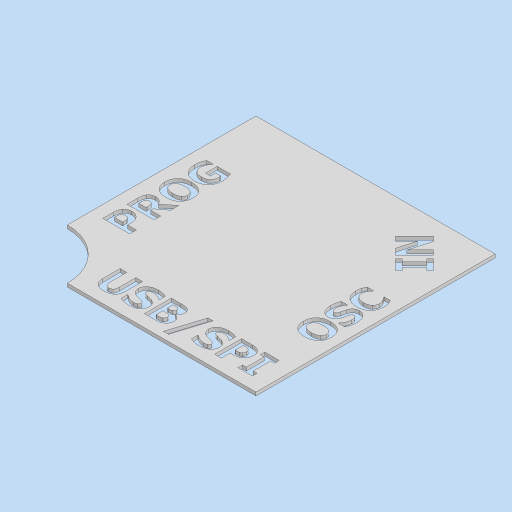
# Autodesk Inventor part: mcu_label
Saved by Autodesk Inventor 2024 (Build 280153000, 153)
## iProperties
Created: 2025-05-08
Part Number: mcu_label
Material: Generic
Document SubType Name: Modeling
Designer: XxPan
Density: 1 g/cm^3
Appearance: Default
Author: XxPan
Autodesk Inventor part; units mm, degrees
ref_plane "YZ Plane" through (0, 0, 0) normal (1, 0, 0) x (0, 1, 0)
ref_plane "XZ Plane" through (0, 0, 0) normal (0, 1, 0) x (-1, 0, 0)
ref_plane "XY Plane" through (0, 0, 0) normal (0, 0, 1) x (1, 0, 0)
sketch "Sketch1" plane through (0, 0, 0) normal (0, 1, 0) x (-1, 0, 0)
  line L0 (0, 0) -> (7.1, 0)
  line L1 (7.1, 0) -> (7.1, -7.1)
  line L2 (7.1, -7.1) -> (0, -7.1)
  line L3 (0, -7.1) -> (0, 0)
  dimension "d0" = 7.1
  dimension "d1" = 7.1
  constraints: 8 end point, 2 parallel, 1 horizontal, 1 perpendicular
  measures "d0" distance of L1.end L2.end
  measures "d1" distance of L0.end L1.end
extrude "Extrusion1" add sketch "Sketch1" along normal blind 0.1
fillet "Fillet1" radius 1.5 1 edges at (-7.1, 0.05, 0) inverted yes
sketch "Sketch2" plane through (0, 0.1, 0) normal (0, 1, 0) x (1, 0, 0)
  line L0 (-6.7596, 2.1096) -> (-6.7596, 12.4131) construction
  line L1 (-6.7596, 12.4131) -> (-3.5966, 12.4131) construction
  line L2 (-3.5966, 12.4131) -> (-3.5966, 2.1096) construction
  line L3 (-3.5966, 2.1096) -> (-6.7596, 2.1096) construction
  line L4 (-1.1207, 2.1079) -> (-1.1207, 12.4115) construction
  line L5 (-1.1207, 12.4115) -> (2.0423, 12.4115) construction
  line L6 (2.0423, 12.4115) -> (2.0423, 2.1079) construction
  line L7 (2.0423, 2.1079) -> (-1.1207, 2.1079) construction
  line L8 (-1.0199, 5.1592) -> (-8.3056, 12.4449) construction
  line L9 (-8.3056, 12.4449) -> (-6.069, 14.6814) construction
  line L10 (-6.069, 14.6814) -> (1.2167, 7.3958) construction
  line L11 (1.2167, 7.3958) -> (-1.0199, 5.1592) construction
  line L12 (-5.2671, -1.9674) -> (-5.2671, 1.1956) construction
  line L13 (-5.2671, 1.1956) -> (5.0364, 1.1956) construction
  line L14 (5.0364, 1.1956) -> (5.0364, -1.9674) construction
  line L15 (5.0364, -1.9674) -> (-5.2671, -1.9674) construction
  spline S0 degree 2 poles (-4.8607, 0.343) (-5.0221, 0.343) (-5.1958, 0.4986) (-5.1958, 0.649) knots 0 0 0 1 2 2 2
  line L16 (-5.1958, 0.649) -> (-5.1958, 1.1599)
  line L17 (-5.1958, 1.1599) -> (-4.9949, 1.1599)
  line L18 (-4.9949, 1.1599) -> (-4.9949, 0.6607)
  spline S1 degree 2 poles (-4.9949, 0.6607) (-4.9949, 0.5771) (-4.932, 0.4954) (-4.8607, 0.4954) knots 0 0 0 1 2 2 2
  spline S2 degree 2 poles (-4.8607, 0.4954) (-4.7913, 0.4954) (-4.7265, 0.5738) (-4.7265, 0.6607) knots 0 0 0 1 2 2 2
  line L19 (-4.7265, 0.6607) -> (-4.7265, 1.1599)
  line L20 (-4.7265, 1.1599) -> (-4.5255, 1.1599)
  line L21 (-4.5255, 1.1599) -> (-4.5255, 0.6497)
  spline S3 degree 2 poles (-4.5255, 0.6497) (-4.5255, 0.5019) (-4.6947, 0.343) (-4.8607, 0.343) knots 0 0 0 1 2 2 2
  spline S4 degree 2 poles (-4.1242, 0.3456) (-4.2163, 0.3456) (-4.355, 0.3813) (-4.4146, 0.4072) knots 0 0 0 1 2 2 2
  line L22 (-4.4146, 0.4072) -> (-4.4146, 0.5978)
  line L23 (-4.4146, 0.5978) -> (-4.3965, 0.5978)
  spline S5 degree 2 poles (-4.3965, 0.5978) (-4.3362, 0.5466) (-4.1916, 0.4915) (-4.1235, 0.4915) knots 0 0 0 1 2 2 2
  spline S6 degree 2 poles (-4.1235, 0.4915) (-4.106, 0.4915) (-4.0496, 0.4993) (-4.0328, 0.5071) knots 0 0 0 1 2 2 2
  spline S7 degree 2 poles (-4.0328, 0.5071) (-4.012, 0.5161) (-3.9829, 0.5492) (-3.9829, 0.5758) knots 0 0 0 1 2 2 2
  spline S8 degree 2 poles (-3.9829, 0.5758) (-3.9829, 0.6063) (-4.0302, 0.6439) (-4.0626, 0.6523) knots 0 0 0 1 2 2 2
  spline S9 degree 2 poles (-4.0626, 0.6523) (-4.1034, 0.6633) (-4.1962, 0.6821) (-4.237, 0.6964) knots 0 0 0 1 2 2 2
  spline S10 degree 2 poles (-4.237, 0.6964) (-4.3297, 0.7288) (-4.4101, 0.8396) (-4.4101, 0.9226) knots 0 0 0 1 2 2 2
  spline S11 degree 2 poles (-4.4101, 0.9226) (-4.4101, 1.0348) (-4.2201, 1.1742) (-4.0775, 1.1742) knots 0 0 0 1 2 2 2
  spline S12 degree 2 poles (-4.0775, 1.1742) (-4.0062, 1.1742) (-3.8649, 1.145) (-3.8091, 1.1204) knots 0 0 0 1 2 2 2
  line L24 (-3.8091, 1.1204) -> (-3.8091, 0.9375)
  line L25 (-3.8091, 0.9375) -> (-3.8266, 0.9375)
  spline S13 degree 2 poles (-3.8266, 0.9375) (-3.8714, 0.9758) (-3.9997, 1.0283) (-4.0671, 1.0283) knots 0 0 0 1 2 2 2
  spline S14 degree 2 poles (-4.0671, 1.0283) (-4.0937, 1.0283) (-4.1352, 1.0205) (-4.1586, 1.0101) knots 0 0 0 1 2 2 2
  spline S15 degree 2 poles (-4.1586, 1.0101) (-4.1774, 1.0017) (-4.2046, 0.968) (-4.2046, 0.9473) knots 0 0 0 1 2 2 2
  spline S16 degree 2 poles (-4.2046, 0.9473) (-4.2046, 0.9161) (-4.1611, 0.8805) (-4.0989, 0.8662) knots 0 0 0 1 2 2 2
  spline S17 degree 2 poles (-4.0989, 0.8662) (-4.0587, 0.8571) (-3.9842, 0.8396) (-3.9414, 0.8247) knots 0 0 0 1 2 2 2
  spline S18 degree 2 poles (-3.9414, 0.8247) (-3.8584, 0.7943) (-3.7774, 0.6931) (-3.7774, 0.6101) knots 0 0 0 1 2 2 2
  spline S19 degree 2 poles (-3.7774, 0.6101) (-3.7774, 0.4909) (-3.9647, 0.3456) (-4.1242, 0.3456) knots 0 0 0 1 2 2 2
  spline S20 degree 2 poles (-3.0351, 0.605) (-3.0351, 0.5453) (-3.0804, 0.4552) (-3.118, 0.4254) knots 0 0 0 1 2 2 2
  spline S21 degree 2 poles (-3.118, 0.4254) (-3.1634, 0.3897) (-3.271, 0.3599) (-3.3547, 0.3599) knots 0 0 0 1 2 2 2
  line L26 (-3.3547, 0.3599) -> (-3.6743, 0.3599)
  line L27 (-3.6743, 0.3599) -> (-3.6743, 1.1599)
  line L28 (-3.6743, 1.1599) -> (-3.3923, 1.1599)
  spline S22 degree 2 poles (-3.3923, 1.1599) (-3.3041, 1.1599) (-3.2133, 1.1463) (-3.1738, 1.1249) knots 0 0 0 1 2 2 2
  spline S23 degree 2 poles (-3.1738, 1.1249) (-3.1304, 1.1022) (-3.0882, 1.0244) (-3.0882, 0.9738) knots 0 0 0 1 2 2 2
  spline S24 degree 2 poles (-3.0882, 0.9738) (-3.0882, 0.9155) (-3.1466, 0.8241) (-3.1984, 0.8027) knots 0 0 0 1 2 2 2
  line L29 (-3.1984, 0.8027) -> (-3.1984, 0.7988)
  spline S25 degree 2 poles (-3.1984, 0.7988) (-3.1239, 0.7832) (-3.0351, 0.6866) (-3.0351, 0.605) knots 0 0 0 1 2 2 2
  spline S26 degree 2 poles (-3.2425, 0.6082) (-3.2425, 0.6458) (-3.2723, 0.6879) (-3.3022, 0.699) knots 0 0 0 1 2 2 2
  spline S27 degree 2 poles (-3.3022, 0.699) (-3.3203, 0.7061) (-3.3845, 0.7074) (-3.4376, 0.7074) knots 0 0 0 1 2 2 2
  line L30 (-3.4376, 0.7074) -> (-3.4746, 0.7074)
  line L31 (-3.4746, 0.7074) -> (-3.4746, 0.5058)
  line L32 (-3.4746, 0.5058) -> (-3.4636, 0.5058)
  spline S28 degree 2 poles (-3.4636, 0.5058) (-3.3858, 0.5058) (-3.3261, 0.5077) (-3.295, 0.5213) knots 0 0 0 1 2 2 2
  spline S29 degree 2 poles (-3.295, 0.5213) (-3.2678, 0.5336) (-3.2425, 0.579) (-3.2425, 0.6082) knots 0 0 0 1 2 2 2
  spline S30 degree 2 poles (-3.2924, 0.9343) (-3.2924, 0.9537) (-3.3125, 0.9946) (-3.3333, 1.0037) knots 0 0 0 1 2 2 2
  spline S31 degree 2 poles (-3.3333, 1.0037) (-3.3527, 1.0127) (-3.4072, 1.014) (-3.461, 1.014) knots 0 0 0 1 2 2 2
  line L33 (-3.461, 1.014) -> (-3.4746, 1.014)
  line L34 (-3.4746, 1.014) -> (-3.4746, 0.8442)
  line L35 (-3.4746, 0.8442) -> (-3.4493, 0.8442)
  spline S32 degree 2 poles (-3.4493, 0.8442) (-3.3981, 0.8442) (-3.3566, 0.8461) (-3.3346, 0.8565) knots 0 0 0 1 2 2 2
  spline S33 degree 2 poles (-3.3346, 0.8565) (-3.3106, 0.8682) (-3.2924, 0.9077) (-3.2924, 0.9343) knots 0 0 0 1 2 2 2
  line L36 (-2.4665, 1.1956) -> (-2.7848, 0.1862)
  line L37 (-2.7848, 0.1862) -> (-2.9391, 0.1862)
  line L38 (-2.9391, 0.1862) -> (-2.6214, 1.1956)
  line L39 (-2.6214, 1.1956) -> (-2.4665, 1.1956)
  spline S34 degree 2 poles (-2.038, 0.3456) (-2.13, 0.3456) (-2.2688, 0.3813) (-2.3284, 0.4072) knots 0 0 0 1 2 2 2
  line L40 (-2.3284, 0.4072) -> (-2.3284, 0.5978)
  line L41 (-2.3284, 0.5978) -> (-2.3103, 0.5978)
  spline S35 degree 2 poles (-2.3103, 0.5978) (-2.25, 0.5466) (-2.1054, 0.4915) (-2.0373, 0.4915) knots 0 0 0 1 2 2 2
  spline S36 degree 2 poles (-2.0373, 0.4915) (-2.0198, 0.4915) (-1.9634, 0.4993) (-1.9466, 0.5071) knots 0 0 0 1 2 2 2
  spline S37 degree 2 poles (-1.9466, 0.5071) (-1.9258, 0.5161) (-1.8966, 0.5492) (-1.8966, 0.5758) knots 0 0 0 1 2 2 2
  spline S38 degree 2 poles (-1.8966, 0.5758) (-1.8966, 0.6063) (-1.944, 0.6439) (-1.9764, 0.6523) knots 0 0 0 1 2 2 2
  spline S39 degree 2 poles (-1.9764, 0.6523) (-2.0172, 0.6633) (-2.1099, 0.6821) (-2.1508, 0.6964) knots 0 0 0 1 2 2 2
  spline S40 degree 2 poles (-2.1508, 0.6964) (-2.2435, 0.7288) (-2.3239, 0.8396) (-2.3239, 0.9226) knots 0 0 0 1 2 2 2
  spline S41 degree 2 poles (-2.3239, 0.9226) (-2.3239, 1.0348) (-2.1339, 1.1742) (-1.9913, 1.1742) knots 0 0 0 1 2 2 2
  spline S42 degree 2 poles (-1.9913, 1.1742) (-1.92, 1.1742) (-1.7787, 1.145) (-1.7229, 1.1204) knots 0 0 0 1 2 2 2
  line L42 (-1.7229, 1.1204) -> (-1.7229, 0.9375)
  line L43 (-1.7229, 0.9375) -> (-1.7404, 0.9375)
  spline S43 degree 2 poles (-1.7404, 0.9375) (-1.7851, 0.9758) (-1.9135, 1.0283) (-1.9809, 1.0283) knots 0 0 0 1 2 2 2
  spline S44 degree 2 poles (-1.9809, 1.0283) (-2.0075, 1.0283) (-2.049, 1.0205) (-2.0723, 1.0101) knots 0 0 0 1 2 2 2
  spline S45 degree 2 poles (-2.0723, 1.0101) (-2.0911, 1.0017) (-2.1184, 0.968) (-2.1184, 0.9473) knots 0 0 0 1 2 2 2
  spline S46 degree 2 poles (-2.1184, 0.9473) (-2.1184, 0.9161) (-2.0749, 0.8805) (-2.0127, 0.8662) knots 0 0 0 1 2 2 2
  spline S47 degree 2 poles (-2.0127, 0.8662) (-1.9725, 0.8571) (-1.8979, 0.8396) (-1.8552, 0.8247) knots 0 0 0 1 2 2 2
  spline S48 degree 2 poles (-1.8552, 0.8247) (-1.7722, 0.7943) (-1.6911, 0.6931) (-1.6911, 0.6101) knots 0 0 0 1 2 2 2
  spline S49 degree 2 poles (-1.6911, 0.6101) (-1.6911, 0.4909) (-1.8785, 0.3456) (-2.038, 0.3456) knots 0 0 0 1 2 2 2
  spline S50 degree 2 poles (-0.9728, 0.9077) (-0.9728, 0.852) (-1.0085, 0.7508) (-1.0415, 0.7171) knots 0 0 0 1 2 2 2
  spline S51 degree 2 poles (-1.0415, 0.7171) (-1.0616, 0.6957) (-1.1109, 0.6607) (-1.1401, 0.6484) knots 0 0 0 1 2 2 2
  spline S52 degree 2 poles (-1.1401, 0.6484) (-1.1699, 0.6361) (-1.2393, 0.6218) (-1.2821, 0.6218) knots 0 0 0 1 2 2 2
  line L44 (-1.2821, 0.6218) -> (-1.3871, 0.6218)
  line L45 (-1.3871, 0.6218) -> (-1.3871, 0.3599)
  line L46 (-1.3871, 0.3599) -> (-1.5881, 0.3599)
  line L47 (-1.5881, 0.3599) -> (-1.5881, 1.1599)
  line L48 (-1.5881, 1.1599) -> (-1.2775, 1.1599)
  spline S53 degree 2 poles (-1.2775, 1.1599) (-1.2088, 1.1599) (-1.1083, 1.1346) (-1.0675, 1.1074) knots 0 0 0 1 2 2 2
  spline S54 degree 2 poles (-1.0675, 1.1074) (-1.0221, 1.0769) (-0.9728, 0.9771) (-0.9728, 0.9077) knots 0 0 0 1 2 2 2
  spline S55 degree 2 poles (-1.179, 0.9025) (-1.179, 0.9369) (-1.2114, 0.9855) (-1.2334, 0.9946) knots 0 0 0 1 2 2 2
  spline S56 degree 2 poles (-1.2334, 0.9946) (-1.262, 1.0069) (-1.3138, 1.0108) (-1.3586, 1.0108) knots 0 0 0 1 2 2 2
  line L49 (-1.3586, 1.0108) -> (-1.3871, 1.0108)
  line L50 (-1.3871, 1.0108) -> (-1.3871, 0.7709)
  line L51 (-1.3871, 0.7709) -> (-1.3728, 0.7709)
  spline S57 degree 2 poles (-1.3728, 0.7709) (-1.3449, 0.7709) (-1.2944, 0.7722) (-1.2756, 0.7755) knots 0 0 0 1 2 2 2
  spline S58 degree 2 poles (-1.2756, 0.7755) (-1.2594, 0.7781) (-1.2237, 0.7936) (-1.214, 0.8033) knots 0 0 0 1 2 2 2
  spline S59 degree 2 poles (-1.214, 0.8033) (-1.1932, 0.8228) (-1.179, 0.8662) (-1.179, 0.9025) knots 0 0 0 1 2 2 2
  line L52 (-0.4671, 0.3599) -> (-0.8976, 0.3599)
  line L53 (-0.8976, 0.3599) -> (-0.8976, 0.4993)
  line L54 (-0.8976, 0.4993) -> (-0.7829, 0.4993)
  line L55 (-0.7829, 0.4993) -> (-0.7829, 1.0205)
  line L56 (-0.7829, 1.0205) -> (-0.8976, 1.0205)
  line L57 (-0.8976, 1.0205) -> (-0.8976, 1.1599)
  line L58 (-0.8976, 1.1599) -> (-0.4671, 1.1599)
  line L59 (-0.4671, 1.1599) -> (-0.4671, 1.0205)
  line L60 (-0.4671, 1.0205) -> (-0.5819, 1.0205)
  line L61 (-0.5819, 1.0205) -> (-0.5819, 0.4993)
  line L62 (-0.5819, 0.4993) -> (-0.4671, 0.4993)
  line L63 (-0.4671, 0.4993) -> (-0.4671, 0.3599)
  spline S60 degree 2 poles (-6.4906, 2.8078) (-6.4348, 2.8078) (-6.3337, 2.7722) (-6.3, 2.7391) knots 0 0 0 1 2 2 2
  spline S61 degree 2 poles (-6.3, 2.7391) (-6.2786, 2.719) (-6.2436, 2.6697) (-6.2312, 2.6405) knots 0 0 0 1 2 2 2
  spline S62 degree 2 poles (-6.2312, 2.6405) (-6.2189, 2.6107) (-6.2047, 2.5414) (-6.2047, 2.4986) knots 0 0 0 1 2 2 2
  line L64 (-6.2047, 2.4986) -> (-6.2047, 2.3935)
  line L65 (-6.2047, 2.3935) -> (-5.9428, 2.3935)
  line L66 (-5.9428, 2.3935) -> (-5.9428, 2.1926)
  line L67 (-5.9428, 2.1926) -> (-6.7428, 2.1926)
  line L68 (-6.7428, 2.1926) -> (-6.7428, 2.5031)
  spline S63 degree 2 poles (-6.7428, 2.5031) (-6.7428, 2.5718) (-6.7175, 2.6723) (-6.6902, 2.7132) knots 0 0 0 1 2 2 2
  spline S64 degree 2 poles (-6.6902, 2.7132) (-6.6598, 2.7585) (-6.5599, 2.8078) (-6.4906, 2.8078) knots 0 0 0 1 2 2 2
  spline S65 degree 2 poles (-6.4854, 2.6017) (-6.5197, 2.6017) (-6.5684, 2.5692) (-6.5774, 2.5472) knots 0 0 0 1 2 2 2
  spline S66 degree 2 poles (-6.5774, 2.5472) (-6.5898, 2.5187) (-6.5936, 2.4668) (-6.5936, 2.4221) knots 0 0 0 1 2 2 2
  line L69 (-6.5936, 2.4221) -> (-6.5936, 2.3935)
  line L70 (-6.5936, 2.3935) -> (-6.3538, 2.3935)
  line L71 (-6.3538, 2.3935) -> (-6.3538, 2.4078)
  spline S67 degree 2 poles (-6.3538, 2.4078) (-6.3538, 2.4357) (-6.3551, 2.4863) (-6.3583, 2.5051) knots 0 0 0 1 2 2 2
  spline S68 degree 2 poles (-6.3583, 2.5051) (-6.3609, 2.5213) (-6.3765, 2.5569) (-6.3862, 2.5666) knots 0 0 0 1 2 2 2
  spline S69 degree 2 poles (-6.3862, 2.5666) (-6.4056, 2.5874) (-6.4491, 2.6017) (-6.4854, 2.6017) knots 0 0 0 1 2 2 2
  line L72 (-5.9428, 3.6545) -> (-5.9428, 3.4101)
  line L73 (-5.9428, 3.4101) -> (-6.2364, 3.1877)
  line L74 (-6.2364, 3.1877) -> (-6.2364, 3.1151)
  line L75 (-6.2364, 3.1151) -> (-5.9428, 3.1151)
  line L76 (-5.9428, 3.1151) -> (-5.9428, 2.9154)
  line L77 (-5.9428, 2.9154) -> (-6.7428, 2.9154)
  line L78 (-6.7428, 2.9154) -> (-6.7428, 3.237)
  spline S70 degree 2 poles (-6.7428, 3.237) (-6.7428, 3.3038) (-6.7259, 3.4023) (-6.7, 3.4444) knots 0 0 0 1 2 2 2
  spline S71 degree 2 poles (-6.7, 3.4444) (-6.6727, 3.4872) (-6.5878, 3.5378) (-6.523, 3.5378) knots 0 0 0 1 2 2 2
  spline S72 degree 2 poles (-6.523, 3.5378) (-6.4316, 3.5378) (-6.3168, 3.4548) (-6.2831, 3.3854) knots 0 0 0 1 2 2 2
  line L79 (-6.2831, 3.3854) -> (-5.9428, 3.6545)
  spline S73 degree 2 poles (-6.4977, 3.3316) (-6.5282, 3.3316) (-6.5716, 3.3083) (-6.5833, 3.2817) knots 0 0 0 1 2 2 2
  spline S74 degree 2 poles (-6.5833, 3.2817) (-6.5911, 3.2629) (-6.5956, 3.2169) (-6.5956, 3.1825) knots 0 0 0 1 2 2 2
  line L80 (-6.5956, 3.1825) -> (-6.5956, 3.1151)
  line L81 (-6.5956, 3.1151) -> (-6.3804, 3.1151)
  line L82 (-6.3804, 3.1151) -> (-6.3804, 3.1728)
  spline S75 degree 2 poles (-6.3804, 3.1728) (-6.3804, 3.2143) (-6.3907, 3.2733) (-6.4069, 3.2934) knots 0 0 0 1 2 2 2
  spline S76 degree 2 poles (-6.4069, 3.2934) (-6.4225, 3.3128) (-6.464, 3.3316) (-6.4977, 3.3316) knots 0 0 0 1 2 2 2
  spline S77 degree 2 poles (-6.3428, 4.4422) (-6.1483, 4.4422) (-5.9259, 4.2347) (-5.9259, 4.0545) knots 0 0 0 1 2 2 2
  spline S78 degree 2 poles (-5.9259, 4.0545) (-5.9259, 3.8736) (-6.1509, 3.6675) (-6.3428, 3.6675) knots 0 0 0 1 2 2 2
  spline S79 degree 2 poles (-6.3428, 3.6675) (-6.5353, 3.6675) (-6.7596, 3.8736) (-6.7596, 4.0545) knots 0 0 0 1 2 2 2
  spline S80 degree 2 poles (-6.7596, 4.0545) (-6.7596, 4.2347) (-6.5366, 4.4422) (-6.3428, 4.4422) knots 0 0 0 1 2 2 2
  spline S81 degree 2 poles (-6.3428, 4.2347) (-6.4147, 4.2347) (-6.5152, 4.2055) (-6.547, 4.1803) knots 0 0 0 1 2 2 2
  spline S82 degree 2 poles (-6.547, 4.1803) (-6.58, 4.155) (-6.6086, 4.0901) (-6.6086, 4.0551) knots 0 0 0 1 2 2 2
  spline S83 degree 2 poles (-6.6086, 4.0551) (-6.6086, 4.0182) (-6.582, 3.9579) (-6.5483, 3.93) knots 0 0 0 1 2 2 2
  spline S84 degree 2 poles (-6.5483, 3.93) (-6.5171, 3.9054) (-6.4141, 3.8749) (-6.3428, 3.8749) knots 0 0 0 1 2 2 2
  spline S85 degree 2 poles (-6.3428, 3.8749) (-6.2688, 3.8749) (-6.1716, 3.9041) (-6.1385, 3.9294) knots 0 0 0 1 2 2 2
  spline S86 degree 2 poles (-6.1385, 3.9294) (-6.1055, 3.9546) (-6.077, 4.0201) (-6.077, 4.0551) knots 0 0 0 1 2 2 2
  spline S87 degree 2 poles (-6.077, 4.0551) (-6.077, 4.0908) (-6.1074, 4.1569) (-6.1398, 4.1809) knots 0 0 0 1 2 2 2
  spline S88 degree 2 poles (-6.1398, 4.1809) (-6.1748, 4.2068) (-6.2676, 4.2347) (-6.3428, 4.2347) knots 0 0 0 1 2 2 2
  spline S89 degree 2 poles (-5.9881, 5.2292) (-5.9667, 5.1767) (-5.9259, 5.0088) (-5.9259, 4.9271) knots 0 0 0 1 2 2 2
  spline S90 degree 2 poles (-5.9259, 4.9271) (-5.9259, 4.7384) (-6.1437, 4.5148) (-6.3434, 4.5148) knots 0 0 0 1 2 2 2
  spline S91 degree 2 poles (-6.3434, 4.5148) (-6.5314, 4.5148) (-6.7583, 4.7384) (-6.7583, 4.9329) knots 0 0 0 1 2 2 2
  spline S92 degree 2 poles (-6.7583, 4.9329) (-6.7583, 5.0334) (-6.7201, 5.1592) (-6.6876, 5.226) knots 0 0 0 1 2 2 2
  line L83 (-6.6876, 5.226) -> (-6.4996, 5.226)
  line L84 (-6.4996, 5.226) -> (-6.4996, 5.2078)
  spline S93 degree 2 poles (-6.4996, 5.2078) (-6.5107, 5.1935) (-6.5528, 5.1391) (-6.5671, 5.1132) knots 0 0 0 1 2 2 2
  spline S94 degree 2 poles (-6.5671, 5.1132) (-6.5846, 5.0833) (-6.6092, 5.0042) (-6.6092, 4.9602) knots 0 0 0 1 2 2 2
  spline S95 degree 2 poles (-6.6092, 4.9602) (-6.6092, 4.9089) (-6.5768, 4.824) (-6.5437, 4.791) knots 0 0 0 1 2 2 2
  spline S96 degree 2 poles (-6.5437, 4.791) (-6.5113, 4.7592) (-6.4121, 4.7222) (-6.3466, 4.7222) knots 0 0 0 1 2 2 2
  spline S97 degree 2 poles (-6.3466, 4.7222) (-6.2066, 4.7222) (-6.0731, 4.8629) (-6.0731, 4.9841) knots 0 0 0 1 2 2 2
  spline S98 degree 2 poles (-6.0731, 4.9841) (-6.0731, 4.9952) (-6.0744, 5.0237) (-6.075, 5.0347) knots 0 0 0 1 2 2 2
  line L85 (-6.075, 5.0347) -> (-6.2325, 5.0347)
  line L86 (-6.2325, 5.0347) -> (-6.2325, 4.8798)
  line L87 (-6.2325, 4.8798) -> (-6.3823, 4.8798)
  line L88 (-6.3823, 4.8798) -> (-6.3823, 5.2292)
  line L89 (-6.3823, 5.2292) -> (-5.9881, 5.2292)
  spline S99 degree 2 poles (-0.7038, 2.919) (-0.5093, 2.919) (-0.287, 2.7115) (-0.287, 2.5313) knots 0 0 0 1 2 2 2
  spline S100 degree 2 poles (-0.287, 2.5313) (-0.287, 2.3504) (-0.5119, 2.1443) (-0.7038, 2.1443) knots 0 0 0 1 2 2 2
  spline S101 degree 2 poles (-0.7038, 2.1443) (-0.8964, 2.1443) (-1.1207, 2.3504) (-1.1207, 2.5313) knots 0 0 0 1 2 2 2
  spline S102 degree 2 poles (-1.1207, 2.5313) (-1.1207, 2.7115) (-0.8977, 2.919) (-0.7038, 2.919) knots 0 0 0 1 2 2 2
  spline S103 degree 2 poles (-0.7038, 2.7115) (-0.7758, 2.7115) (-0.8763, 2.6823) (-0.908, 2.6571) knots 0 0 0 1 2 2 2
  spline S104 degree 2 poles (-0.908, 2.6571) (-0.9411, 2.6318) (-0.9696, 2.5669) (-0.9696, 2.5319) knots 0 0 0 1 2 2 2
  spline S105 degree 2 poles (-0.9696, 2.5319) (-0.9696, 2.495) (-0.9431, 2.4347) (-0.9093, 2.4068) knots 0 0 0 1 2 2 2
  spline S106 degree 2 poles (-0.9093, 2.4068) (-0.8782, 2.3822) (-0.7751, 2.3517) (-0.7038, 2.3517) knots 0 0 0 1 2 2 2
  spline S107 degree 2 poles (-0.7038, 2.3517) (-0.6299, 2.3517) (-0.5327, 2.3809) (-0.4996, 2.4062) knots 0 0 0 1 2 2 2
  spline S108 degree 2 poles (-0.4996, 2.4062) (-0.4666, 2.4315) (-0.438, 2.4969) (-0.438, 2.5319) knots 0 0 0 1 2 2 2
  spline S109 degree 2 poles (-0.438, 2.5319) (-0.438, 2.5676) (-0.4685, 2.6337) (-0.5009, 2.6577) knots 0 0 0 1 2 2 2
  spline S110 degree 2 poles (-0.5009, 2.6577) (-0.5359, 2.6836) (-0.6286, 2.7115) (-0.7038, 2.7115) knots 0 0 0 1 2 2 2
  spline S111 degree 2 poles (-0.2896, 3.2853) (-0.2896, 3.1932) (-0.3252, 3.0545) (-0.3512, 2.9948) knots 0 0 0 1 2 2 2
  line L90 (-0.3512, 2.9948) -> (-0.5418, 2.9948)
  line L91 (-0.5418, 2.9948) -> (-0.5418, 3.013)
  spline S112 degree 2 poles (-0.5418, 3.013) (-0.4905, 3.0733) (-0.4354, 3.2178) (-0.4354, 3.2859) knots 0 0 0 1 2 2 2
  spline S113 degree 2 poles (-0.4354, 3.2859) (-0.4354, 3.3034) (-0.4432, 3.3598) (-0.451, 3.3767) knots 0 0 0 1 2 2 2
  spline S114 degree 2 poles (-0.451, 3.3767) (-0.4601, 3.3974) (-0.4931, 3.4266) (-0.5197, 3.4266) knots 0 0 0 1 2 2 2
  spline S115 degree 2 poles (-0.5197, 3.4266) (-0.5502, 3.4266) (-0.5878, 3.3793) (-0.5962, 3.3468) knots 0 0 0 1 2 2 2
  spline S116 degree 2 poles (-0.5962, 3.3468) (-0.6072, 3.306) (-0.626, 3.2133) (-0.6403, 3.1725) knots 0 0 0 1 2 2 2
  spline S117 degree 2 poles (-0.6403, 3.1725) (-0.6727, 3.0797) (-0.7836, 2.9994) (-0.8666, 2.9994) knots 0 0 0 1 2 2 2
  spline S118 degree 2 poles (-0.8666, 2.9994) (-0.9787, 2.9994) (-1.1181, 3.1893) (-1.1181, 3.3319) knots 0 0 0 1 2 2 2
  spline S119 degree 2 poles (-1.1181, 3.3319) (-1.1181, 3.4032) (-1.0889, 3.5446) (-1.0643, 3.6003) knots 0 0 0 1 2 2 2
  line L92 (-1.0643, 3.6003) -> (-0.8815, 3.6003)
  line L93 (-0.8815, 3.6003) -> (-0.8815, 3.5828)
  spline S120 degree 2 poles (-0.8815, 3.5828) (-0.9197, 3.5381) (-0.9722, 3.4097) (-0.9722, 3.3423) knots 0 0 0 1 2 2 2
  spline S121 degree 2 poles (-0.9722, 3.3423) (-0.9722, 3.3157) (-0.9644, 3.2742) (-0.9541, 3.2509) knots 0 0 0 1 2 2 2
  spline S122 degree 2 poles (-0.9541, 3.2509) (-0.9456, 3.2321) (-0.9119, 3.2049) (-0.8912, 3.2049) knots 0 0 0 1 2 2 2
  spline S123 degree 2 poles (-0.8912, 3.2049) (-0.8601, 3.2049) (-0.8244, 3.2483) (-0.8102, 3.3105) knots 0 0 0 1 2 2 2
  spline S124 degree 2 poles (-0.8102, 3.3105) (-0.8011, 3.3507) (-0.7836, 3.4253) (-0.7687, 3.4681) knots 0 0 0 1 2 2 2
  spline S125 degree 2 poles (-0.7687, 3.4681) (-0.7382, 3.5511) (-0.6371, 3.6321) (-0.5541, 3.6321) knots 0 0 0 1 2 2 2
  spline S126 degree 2 poles (-0.5541, 3.6321) (-0.4348, 3.6321) (-0.2896, 3.4447) (-0.2896, 3.2853) knots 0 0 0 1 2 2 2
  spline S127 degree 2 poles (-0.2883, 4.0801) (-0.2883, 3.8998) (-0.5061, 3.6885) (-0.7032, 3.6885) knots 0 0 0 1 2 2 2
  spline S128 degree 2 poles (-0.7032, 3.6885) (-0.8931, 3.6885) (-1.1194, 3.9005) (-1.1194, 4.0807) knots 0 0 0 1 2 2 2
  spline S129 degree 2 poles (-1.1194, 4.0807) (-1.1194, 4.128) (-1.1084, 4.2045) (-1.0993, 4.2396) knots 0 0 0 1 2 2 2
  spline S130 degree 2 poles (-1.0993, 4.2396) (-1.0909, 4.2668) (-1.063, 4.331) (-1.0526, 4.3511) knots 0 0 0 1 2 2 2
  line L94 (-1.0526, 4.3511) -> (-0.862, 4.3511)
  line L95 (-0.862, 4.3511) -> (-0.862, 4.331)
  spline S131 degree 2 poles (-0.862, 4.331) (-0.875, 4.3161) (-0.9113, 4.272) (-0.9281, 4.2441) knots 0 0 0 1 2 2 2
  spline S132 degree 2 poles (-0.9281, 4.2441) (-0.9456, 4.2162) (-0.9696, 4.1494) (-0.9696, 4.1125) knots 0 0 0 1 2 2 2
  spline S133 degree 2 poles (-0.9696, 4.1125) (-0.9696, 4.0691) (-0.9424, 3.9971) (-0.908, 3.964) knots 0 0 0 1 2 2 2
  spline S134 degree 2 poles (-0.908, 3.964) (-0.8776, 3.9342) (-0.7732, 3.896) (-0.7025, 3.896) knots 0 0 0 1 2 2 2
  spline S135 degree 2 poles (-0.7025, 3.896) (-0.628, 3.896) (-0.5262, 3.9355) (-0.4951, 3.9679) knots 0 0 0 1 2 2 2
  spline S136 degree 2 poles (-0.4951, 3.9679) (-0.4646, 3.999) (-0.438, 4.0755) (-0.438, 4.1138) knots 0 0 0 1 2 2 2
  spline S137 degree 2 poles (-0.438, 4.1138) (-0.438, 4.1533) (-0.4646, 4.2253) (-0.4808, 4.2499) knots 0 0 0 1 2 2 2
  spline S138 degree 2 poles (-0.4808, 4.2499) (-0.497, 4.2772) (-0.5314, 4.318) (-0.545, 4.3329) knots 0 0 0 1 2 2 2
  line L96 (-0.545, 4.3329) -> (-0.545, 4.3511)
  line L97 (-0.545, 4.3511) -> (-0.357, 4.3511)
  spline S139 degree 2 poles (-0.357, 4.3511) (-0.3466, 4.329) (-0.3207, 4.2713) (-0.3116, 4.2402) knots 0 0 0 1 2 2 2
  spline S140 degree 2 poles (-0.3116, 4.2402) (-0.2999, 4.2026) (-0.2883, 4.1371) (-0.2883, 4.0801) knots 0 0 0 1 2 2 2
  line L98 (-0.7943, 6.065) -> (-0.49, 5.7606)
  line L99 (-0.49, 5.7606) -> (-0.5885, 5.6621)
  line L100 (-0.5885, 5.6621) -> (-0.6696, 5.7432)
  line L101 (-0.6696, 5.7432) -> (-1.0382, 5.3747)
  line L102 (-1.0382, 5.3747) -> (-0.9571, 5.2935)
  line L103 (-0.9571, 5.2935) -> (-1.0556, 5.195)
  line L104 (-1.0556, 5.195) -> (-1.36, 5.4993)
  line L105 (-1.36, 5.4993) -> (-1.2615, 5.5979)
  line L106 (-1.2615, 5.5979) -> (-1.1803, 5.5168)
  line L107 (-1.1803, 5.5168) -> (-0.8118, 5.8853)
  line L108 (-0.8118, 5.8853) -> (-0.8929, 5.9665)
  line L109 (-0.8929, 5.9665) -> (-0.7943, 6.065)
  line L110 (-1.3733, 6.644) -> (-1.2367, 6.5074)
  line L111 (-1.2367, 6.5074) -> (-1.4127, 5.895)
  line L112 (-1.4127, 5.895) -> (-1.0185, 6.2892)
  line L113 (-1.0185, 6.2892) -> (-0.8888, 6.1595)
  line L114 (-0.8888, 6.1595) -> (-1.4545, 5.5938)
  line L115 (-1.4545, 5.5938) -> (-1.6287, 5.768)
  line L116 (-1.6287, 5.768) -> (-1.4852, 6.2727)
  line L117 (-1.4852, 6.2727) -> (-1.8093, 5.9486)
  line L118 (-1.8093, 5.9486) -> (-1.939, 6.0783)
  line L119 (-1.939, 6.0783) -> (-1.3733, 6.644)
  point P0 (0, 0)
  constraints: 8 other
emboss "Emboss1" sketch "Sketch2" operation cut depth 1 direction (0, -1, 0)
body "Solid1"
